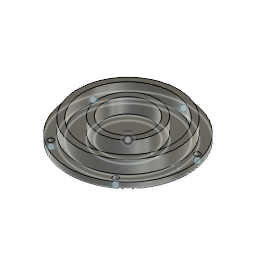
Spinning Tray Assembly (Autodesk Fusion 360 archive; units mm, degrees)
design "Bearing Holder"
part number: 2026-04-22-12-01-27-568
Autodesk Fusion 360 part; units mm, degrees
note: some values were not read from the file. Chosen so that the rebuilt part matches the saved one: which face or edge a step refers to; where a thread starts. Set by a fixed rule: the direction of a hole; which sketch regions a step uses.
sketch "Sketch1" plane through (0, 0, 0) normal (0, 0, 1) x (1, 0, 0)
  circle A0 centre (0, 0) radius 12.75
  circle A1 centre (0, 0) radius 23.95
  circle A2 centre (0, 0) radius 15.75
  circle A3 centre (0, 0) radius 26.95
  circle A4 centre (0, 0) radius 31.95
  circle A5 centre (0.1127, 29.4998) radius 1.5
  circle A6 centre (-28.0211, 9.2231) radius 1.5
  circle A7 centre (-17.4307, -23.7996) radius 1.5
  circle A8 centre (17.2484, -23.9321) radius 1.5
  circle A9 centre (28.0908, 9.0088) radius 1.5
  dimension "d1" = 25.5
  dimension "d3" = 3
  dimension "d4" = 8.2
  dimension "d5" = 3
  dimension "d6" = 5
  dimension "d11" = 3
  dimension "d12" = 29.5
  dimension "d14" = 360
  constraint coincident A0.centre A1.centre
  constraint concentric A0 A1
  constraint concentric A0 A2
  constraint concentric A1 A3
  constraint concentric A3 A4
  measures "d1" diameter of A0
  measures "d3" distance of A0 A2
  measures "d4" distance of A1 A2
  measures "d5" distance of A1 A3
  measures "d6" distance of A3 A4
  measures "d11" diameter of A5
  measures "d12" distance of A0.centre A5.centre
extrude "Extrude1" add sketch "Sketch1" along normal blind 3 contours A0 | A1 | A2 | A3 | A4
extrude "Extrude2" add sketch "Sketch1" along normal blind 10 contours A2 | A3
extrude "Extrude3" add 1 faces at (14.6914, -0.7825, 10) along direction (0, 0, 1) blind 1

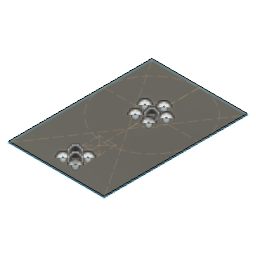
design "Base Plate"
part number: 2026-05-20-10-47-33-993
Autodesk Fusion 360 part; units mm, degrees
sketch "Sketch1" plane through (0, 0, 0) normal (0, 0, 1) x (1, 0, 0)
  line L0 (-71.9661, 43.1181) -> (127.8559, 43.1181)
  line L1 (127.8559, 43.1181) -> (127.8559, -256.8819)
  line L2 (127.8559, -256.8819) -> (-71.9661, -256.8819)
  line L3 (-71.9661, -256.8819) -> (-71.9661, 43.1181)
  line L4 (27.9449, 43.1181) -> (27.9449, -56.8819) construction
  line L5 (-71.9661, -56.8819) -> (127.8559, -56.8819) construction
  line L6 (-71.9661, 43.1181) -> (127.8559, -256.8819) construction
  line L7 (-71.9661, -256.8819) -> (127.8559, 43.1181) construction
  line L8 (27.9449, -106.8819) -> (27.9449, 43.1181) construction
  circle A0 centre (27.9449, -56.8819) radius 31.9337 construction
  circle A1 centre (28.8006, -32.4437) radius 1.5
  circle A2 centre (4.9672, -48.5163) radius 1.5
  circle A3 centre (12.8882, -76.1499) radius 1.5
  circle A4 centre (41.617, -77.1558) radius 1.5
  circle A5 centre (51.4514, -50.1439) radius 1.5
  line L9 (27.9449, -56.8819) -> (27.9449, -216.8819) construction
  circle A6 centre (27.9449, -216.8819) radius 17.5 construction
  line L10 (27.9449, -216.8819) -> (10.4449, -216.8819) construction
  line L11 (27.9449, -216.8819) -> (45.4449, -216.8819) construction
  line L12 (27.9449, -216.8819) -> (27.9449, -199.3819) construction
  line L13 (27.9449, -216.8819) -> (27.9449, -234.3819) construction
  line L14 (45.4449, -216.8819) -> (45.4449, -149.3819) construction
  line L15 (45.4449, -149.3819) -> (10.4449, -149.3819) construction
  line L16 (10.4449, -149.3819) -> (10.4449, -184.3819) construction
  line L17 (10.4449, -184.3819) -> (45.4449, -184.3819) construction
  line L18 (10.4449, -149.3819) -> (45.4449, -184.3819) construction
  line L19 (10.4449, -184.3819) -> (45.4449, -149.3819) construction
  line L20 (27.9449, -216.8819) -> (14.8634, -203.8004) construction
  circle A7 centre (14.8634, -203.8004) radius 1.5
  circle A8 centre (14.8634, -229.9634) radius 1.5
  circle A9 centre (41.0263, -229.9634) radius 1.5
  circle A10 centre (41.0263, -203.8004) radius 1.5
  circle A11 centre (27.9449, -56.8819) radius 100 construction
  dimension "d1" = 199.822
  dimension "d2" = 300
  dimension "d6" = 100
  dimension "d7" = 3
  dimension "d9" = 360
  dimension "d12" = 160
  dimension "d13" = 63.8673
  dimension "d14" = 35
  dimension "d15" = 35
  dimension "d16" = 35
  dimension "d17" = 18.5
  dimension "d18" = 3
  dimension "d20" = 360
  dimension "d23" = 200
  constraint horizontal L0
  constraint vertical L1
  constraint horizontal L2
  constraint vertical L3
  constraint coincident L0 L4.start
  constraint perpendicular L0 L4
  constraint coincident L3 L5.start
  constraint coincident L1 L5.end
  constraint perpendicular L1 L5
  constraint midpoint L7 L8.start
  constraint midpoint L0 L4.start
  constraint midpoint L4.end L5
  constraint coincident L4.end A0.centre
  constraint parallel L8 L9
  constraint coincident L9.end A6.centre
  constraint coincident A6 L10.end
  constraint perpendicular L9 L10
  constraint coincident A6 L11.end
  constraint perpendicular L9 L11
  constraint coincident L9 L12.end
  constraint coincident A6 L12.end
  constraint coincident A6 L13.end
  constraint perpendicular L10 L13
  constraint tangent A6 L14
  constraint perpendicular L12 L15
  constraint perpendicular L10 L16
  constraint perpendicular L13 L17
  constraint perpendicular L18 L19
  constraint perpendicular L19 L20
  constraint coincident L20.end A7.centre
  constraint concentric A0 A11
  measures "d1" distance of L0.start L0.end
  measures "d2" distance of L0.start L2.end
  measures "d6" distance of L4.start L4.end
  measures "d7" diameter of A1
  measures "d12" distance of L4.end L9.end
  measures "d13" diameter of A0
  measures "d14" diameter of A6
  measures "d15" distance of L14.end L15.end
  measures "d16" distance of L15.end L16.end
  measures "d17" distance of L9.end L20.end
  measures "d18" diameter of A7
  measures "d23" diameter of A11
extrude "Extrude1" add sketch "Sketch1" along normal blind 3 contours L0 L1 L2 L3 | A1 | A2 | A3 | A4 | A5 | A7 | A8 | A9 | A10
extrude "Extrude2" cut sketch "Sketch1" along normal blind 17 contours A1 | A2 | A3 | A4 | A5
extrude "Extrude3" cut sketch "Sketch1" along normal blind 23 contours A7 | A8 | A9 | A10

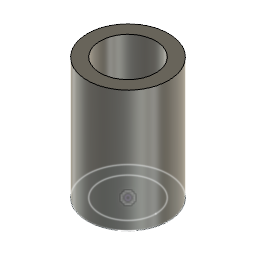
design "SupportBeam'"
part number: 2026-05-20-16-22-24-892
Autodesk Fusion 360 part; units mm, degrees
sketch "Sketch1" plane through (0, 0, 0) normal (0, 0, 1) x (1, 0, 0)
  circle A0 centre (0, 0) radius 6
  circle A1 centre (0, 0) radius 4.1
  dimension "d1" = 12
  dimension "d2" = 8.2
  constraint coincident A0.centre A1.centre
  constraint concentric A0 A1
  measures "d1" diameter of A0
  measures "d2" diameter of A1
extrude "Extrude1" add sketch "Sketch1" along normal blind 18 contours A0 | A1
extrude "Extrude2" cut sketch "Sketch1" against normal blind 7 from surface at 18 contours A1
hole "Hole1" at (0, 0, 0) direction (0, 0, 1) diameter 2.529 depth 10 tip angle 180
thread "Thread1" "ISO Metric profile 3.0 M3x0.5 M3x0.5 6H" major diameter 3.086 minor diameter 2.529 pitch 0.5 angle 60 modelled right hand crest width 0.1368 on face at (0.063, 1.2629, 3.3333) crest through (0, 1.2645, 0)

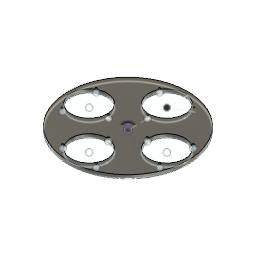
design "Tray Upper Disk"
part number: 2026-04-21-17-23-39-704
Autodesk Fusion 360 part; units mm, degrees
sketch "Sketch1" plane through (0, 0, 0) normal (0, 0, 1) x (1, 0, 0)
  circle A0 centre (0, 0) radius 100
  circle A1 centre (0, 65) radius 30
  circle A2 centre (-65, 0) radius 30
  circle A3 centre (0, -65) radius 30
  circle A4 centre (65, 0) radius 30
  line L0 (0, 65) -> (0, 100) construction
  circle A5 centre (0.1023, 32.5002) radius 1.6
  circle A6 centre (28.0946, 81.3385) radius 1.6
  circle A7 centre (-28.1968, 81.1614) radius 1.6
  circle A8 centre (-32.5002, 0.1023) radius 1.6
  circle A9 centre (-81.1614, -28.1968) radius 1.6
  circle A10 centre (-81.3385, 28.0946) radius 1.6
  circle A11 centre (-0.1023, -32.5002) radius 1.6
  circle A12 centre (28.1968, -81.1614) radius 1.6
  circle A13 centre (-28.0946, -81.3385) radius 1.6
  circle A14 centre (32.5002, -0.1023) radius 1.6
  circle A15 centre (81.1614, 28.1968) radius 1.6
  circle A16 centre (81.3385, -28.0946) radius 1.6
  line L1 (0, 0) -> (0, 100) construction
  line L2 (28.0946, 81.3385) -> (0, 65)
  dimension "d1" = 200
  dimension "d2" = 60
  dimension "d3" = 65
  dimension "d5" = 360
  dimension "d8" = 3.2
  dimension "d9" = 32.5
  dimension "d11" = 360
  dimension "d13" = 360
  constraint coincident A0.centre L1.start
  constraint coincident A1.centre L0.start
  constraint coincident A0 L0.end
  constraint vertical L0
  constraint vertical L1
  constraint coincident A1.centre L1
  constraint coincident A6.centre L2.start
  measures "d1" diameter of A0
  measures "d2" diameter of A1
  measures "d3" distance of A0.centre A1.centre
  measures "d8" diameter of A5
  measures "d9" distance of A1.centre A5.centre
extrude "Extrude1" add sketch "Sketch1" along normal blind 6

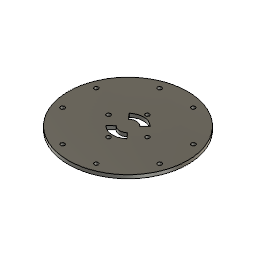
design "Tray Bottom Disk"
part number: 2026-04-21-16-12-52-591
Autodesk Fusion 360 part; units mm, degrees
sketch "Sketch1" plane through (0, 0, 0) normal (0, 0, 1) x (1, 0, 0)
  circle A0 centre (0, 0) radius 100
  circle A1 centre (0, 0) radius 26
  circle A2 centre (0, 0) radius 14
  line L0 (0, 0) -> (17.3974, -19.3218)
  line L1 (0, 0) -> (-26, 0) construction
  line L2 (0, 0) -> (-17.3974, 19.3218)
  line L3 (0, 0) -> (-19.0152, -17.732)
  line L4 (0, 0) -> (19.0152, 17.732)
  line L5 (0, 0) -> (0, 100) construction
  circle A3 centre (0, 32.5) radius 3.35
  line L6 (0, 100) -> (0, 65) construction
  circle A4 centre (28.1458, 81.25) radius 3.35
  circle A5 centre (-28.1458, 81.25) radius 3.35
  circle A6 centre (-32.5, 0) radius 3.35
  circle A7 centre (-81.25, -28.1458) radius 3.35
  circle A8 centre (-81.25, 28.1458) radius 3.35
  circle A9 centre (0, -32.5) radius 3.35
  circle A10 centre (28.1458, -81.25) radius 3.35
  circle A11 centre (-28.1458, -81.25) radius 3.35
  circle A12 centre (32.5, 0) radius 3.35
  circle A13 centre (81.25, 28.1458) radius 3.35
  circle A14 centre (81.25, -28.1458) radius 3.35
  circle A15 centre (0, 0) radius 4.35
  circle A16 centre (0, 65) radius 32.5 construction
  circle A17 centre (0, 65) radius 30 construction
  dimension "d1" = 200
  dimension "d2" = 52
  dimension "d3" = 28
  dimension "d5" = 132
  dimension "d6" = 89
  dimension "d11" = 35
  dimension "d13" = 360
  dimension "d15" = 360
  dimension "d16" = 8.7
  dimension "d17" = 6.7
  dimension "d18" = 65
  dimension "d19" = 60
  constraint coincident A0.centre A1.centre
  constraint concentric A0 A1
  constraint concentric A1 A2
  constraint coincident A1 L0.end
  constraint coincident A1 L1.end
  constraint horizontal L1
  constraint coincident A1 L2.end
  constraint parallel L0 L2
  constraint coincident A1 L3.end
  constraint coincident A1 L4.end
  constraint parallel L3 L4
  constraint coincident A0 L5.end
  constraint vertical L5
  constraint parallel L5 L6
  constraint coincident A3.centre A16
  constraint coincident L5 L6.end
  constraint coincident A5.centre A16
  constraint coincident L5 A3.centre
  constraint coincident L6.end A16.centre
  measures "d1" diameter of A0
  measures "d2" diameter of A1
  measures "d3" diameter of A2
  measures "d5" angle of L0 L1
  measures "d6" angle of L0 L3
  measures "d11" distance of L5.end L6.end
  measures "d16" diameter of A15
  measures "d17" diameter of A3
  measures "d18" diameter of A16
  measures "d19" diameter of A17
extrude "Extrude1" add sketch "Sketch1" along normal blind 6 contours A0 | A1 A2 L0 L4 | A1 A2 L2 L3 | A2 L2 L4 A15 | A2 L0 L4 A15 | A2 L0 L3 A15 | A2 L2 L3 A15 | L0 L4 A15 | L2 L4 A15 | L0 L3 A15 | L2 L3 A15

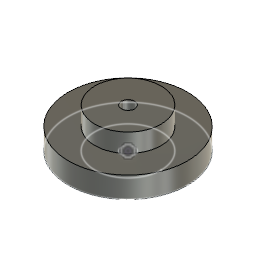
design "Big Pulley"
part number: 2026-04-21-16-11-48-063
Autodesk Fusion 360 part; units mm, degrees
sketch "Sketch2" plane through (0, 0, 0) normal (0, 0, 1) x (1, 0, 0)
  circle A0 centre (0, 0) radius 22.5
  circle A1 centre (0, 0) radius 12.5
  circle A2 centre (0, 0) radius 2.5
  dimension "d1" = 45
  dimension "d2" = 25
  dimension "d3" = 5
  constraint coincident A0.centre A1.centre
  constraint concentric A0 A2
  measures "d1" diameter of A0
  measures "d2" diameter of A1
  measures "d3" diameter of A2
extrude "Extrude1" add sketch "Sketch2" along normal blind 15 contours A1
extrude "Extrude2" add sketch "Sketch2" along normal blind 8 contours A0
